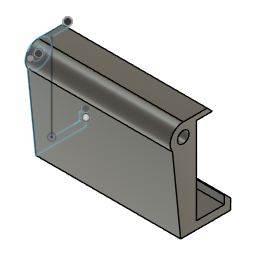
rear plate graber v2 (Autodesk Fusion 360 design; units mm, degrees)
Autodesk Fusion 360 part; units mm, degrees
note: some values were not read from the file. Set by a fixed rule: which sketch regions a step uses.
sketch "Sketch2" plane through (0, 0, 0) normal (1, 0, 0) x (0, 1, 0) in component "rear plate graber"
  line L0 (0, 0) -> (0, 16.5)
  line L1 (3.0285, 16.5) -> (3.0285, 16.5046)
  line L2 (2.0319, 17.512) -> (-1.5, 17.512)
  line L3 (2.0319, 17.512) -> (3.0285, 16.5046)
  line L4 (0, 0) -> (5.3, 0)
  line L5 (6.5, 0) -> (6.4723, -1.5)
  line L6 (6.4723, -1.5) -> (0, -1.5)
  line L7 (4.3, 0) -> (5.3, 0)
  circle A0 centre (-2.5, 15.012) radius 1.1
  line L8 (6.5, 0) -> (6.5, 0.5)
  line L9 (5.5, 1.5) -> (5.3, 1.5)
  line L10 (5.3, 1.5) -> (5.3, 0)
  line L11 (6.5, 0.5) -> (5.5, 1.5)
  line L12 (-2.5, 15.012) -> (-3.4011, 14.3811) construction
  line L13 (-2.5, 15.012) -> (-4.0845, 15.012) construction
  line L14 (0, 16.5) -> (3.0285, 16.5)
  circle A1 centre (-2.5, 15.012) radius 2.5
  line L15 (-1.5, 17.512) -> (-2.5, 17.512)
  line L16 (-4.5479, 13.5781) -> (-3, -1.5)
  line L17 (0, -1.5) -> (-3, -1.5)
  point P0 (3.0319, 17.512)
  point P1 (6.5, 1.5)
  dimension "d4" = 16.5
  dimension "d6" = 1
  dimension "d52" = 2.2
  dimension "d53" = 1.2
  dimension "d54" = 1.5
  dimension "d55" = 1
  dimension "d56" = 1
  dimension "d64" = 35
  dimension "d65" = 5
  constraint coincident L0.start L4.start
  constraint vertical L0
  constraint horizontal L2
  constraint coincident P0 L2
  constraint coincident P0 L1
  constraint horizontal L4
  constraint horizontal L6
  constraint coincident L4 L7.start
  constraint vertical L8
  constraint horizontal L9
  constraint vertical L10
  constraint coincident P1 L8
  constraint coincident P1 L9
  constraint horizontal L13
  constraint coincident A0.centre L12.start
  constraint coincident A0 L12.end
  constraint coincident L0 L4.start
  constraint tangent L0 A1
  constraint tangent L2 A1
  constraint coincident A1 L15.end
  constraint tangent A1 L15
  constraint parallel L2 L15
  constraint coincident A1 L16.start
  measures "d4" distance of L0.start L0.end
  measures "d6" distance of P0 L2.start
  measures "d52" diameter of A0
  measures "d53" distance of L4.end L5.start
  measures "d54" distance of L4.end L9.end
  measures "d55" distance of P1 L8.end
  measures "d56" distance of P1 L9.start
  measures "d64" angle of L12 L13
  measures "d65" diameter of A1
extrude "Extrude2" add sketch "Sketch2" along normal blind 27.5 contours L0 L4 L5 L6 L7 L8 L9 L10 L11 A1 L16 L17 | L0 L1 L2 L3 L14 A1 L15 in component "rear plate graber"
sketch "Sketch4" plane through (0, 0, 0) normal (0, 1, 0) x (-1, 0, 0) in component "rear plate graber"
  line L0 (0, 0) -> (0, 15.012)
  line L1 (0, 16.5) -> (-27.5, 16.5)
  line L2 (-27.5, 15.012) -> (-27.5, 0)
  line L3 (-27.5, 0) -> (0, 0)
  line L4 (-19, 3) -> (-5.5, 3) construction
  line L5 (-5.5, 3) -> (-5.5, 9) construction
  line L6 (-5.5, 9) -> (-19, 9) construction
  line L7 (-19, 9) -> (-19, 3) construction
  line L8 (0, 15.012) -> (0, 16.5)
  line L9 (-27.5, 16.5) -> (-27.5, 15.012)
  line L10 (-27.5, 15.012) -> (0, 15.012)
  line L11 (0, 15.012) -> (-27.5, 15.012)
  dimension "d35" = 3.5
  text T0 "1.0\n" font "Arial" height 3.5 align left top in box 13.5 x 6 at (-19, 3) x (1, 0) y (0, 1) spacing 1
extrude "Extrude4" cut sketch "Sketch4" against normal blind 0.5 text T0 in component "rear plate graber"
extrude "Extrude8" add sketch "Sketch2" along normal blind 27.5 contours A1 in component "rear plate graber"
component "rear plate graber" placed x (1, 0, 0) y (0, 1, 0) z (0, 0, 1) at (0, 0, 0)
equation "d56 = d55"
